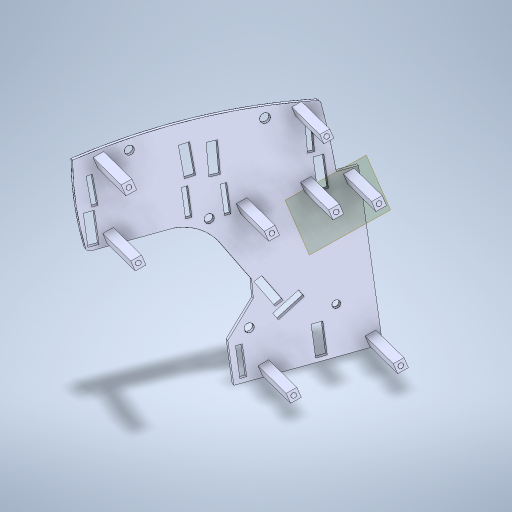
# Autodesk Inventor part: Back Locking Plate - Copy
Saved by Autodesk Inventor 2023 (Build 270158000, 158)
## iProperties
Created: 2022-06-21
Part Number: Back Locking Plate - Copy
Material: Generic
Document SubType Name: Modeling
Designer: Viking Robotics
Density: 1 g/cm^3
Appearance: Default
Sending System: SolidWorks 2019
Last Author: Mahdi
Last Saved: 2022-06-22
Nomenclature: Locking Plate^Bionic Hand
Part Number: Locking Plate^Bionic Hand
Source: NOT_KNOWN
Definition: UNKNOWN
Author: Viking Robotics
Revision Number: ANY
Autodesk Inventor part; units mm, degrees
ref_plane "YZ Plane" through (0, 0, 0) normal (1, 0, 0) x (0, 1, 0)
ref_plane "XZ Plane" through (0, 0, 0) normal (0, 1, 0) x (-1, 0, 0)
ref_plane "XY Plane" through (0, 0, 0) normal (0, 0, 1) x (1, 0, 0)
ref_plane "Work Plane1" through (33.7996, 98.7584, 64.8553) normal (-0.8982078, -0.208723, -0.3868559) x (-0.3186618, -0.2970233, 0.9001288)
sketch "Sketch1" plane through (33.7996, 98.7584, 64.8553) normal (-0.8982078, -0.208723, -0.3868559) x (-0.3186618, -0.2970233, 0.9001288)
  arc A0 (-7.7797, 37.2562) -> (-8.548, 35.9468) centre (-7.048, 35.9468) ccw projected
  arc A1 (73.401, 61.9277) -> (-7.7797, 37.2562) centre (99.9054, -171.1811) ccw
  arc A2 (81.3006, 30.494) -> (73.401, 61.9277) centre (-35.2667, 17.9089) ccw
  arc A3 (-7.7797, 37.2562) -> (-8.548, 35.9468) centre (-7.048, 35.9468) ccw
  arc A4 (-8.548, 35.9468) -> (10.4046, -36.8802) centre (326.4078, 84.2366) ccw
  line L0 (15.9733, -35.39) -> (12.1475, -36.4138) projected
  line L1 (10.4046, -36.8802) -> (15.9733, -35.39)
  line L2 (19.5666, -48.8176) -> (15.9733, -35.39) projected
  line L3 (15.9733, -35.39) -> (19.5666, -48.8176)
  line L4 (55.0191, -39.3303) -> (19.5666, -48.8176) projected
  line L5 (19.5666, -48.8176) -> (55.0191, -39.3303)
  line L6 (37.6609, -14.8207) -> (50.8667, -23.8132) projected
  line L7 (55.0191, -39.3303) -> (50.8667, -23.8132)
  line L8 (50.8667, -23.8132) -> (37.6609, -14.8207)
  line L9 (35.6144, -8.3962) -> (37.6609, -14.8207) projected
  line L10 (37.6609, -14.8207) -> (35.6144, -8.3962)
  line L11 (40.4472, 9.6168) -> (35.6144, -8.3962) projected
  line L12 (35.6144, -8.3962) -> (40.4472, 9.6168)
  arc A5 (52.2969, 22.0311) -> (40.4472, 9.6168) centre (58.9658, 3.8029) ccw
  line L13 (52.2969, 22.0311) -> (79.8228, 29.4185)
  arc A6 (79.8228, 29.4185) -> (81.3006, 31.4948) centre (79.3058, 31.3505) ccw projected
  arc A7 (79.8228, 29.4185) -> (81.3006, 30.494) centre (78.5946, 32.659) ccw
  line L14 (-3.3432, 32.1166) -> (-1.249, 32.7909) projected
  line L15 (-3.3432, 32.1166) -> (-1.249, 32.7909)
  line L16 (-1.249, 32.7909) -> (2.1836, 22.1298)
  line L17 (2.1836, 22.1298) -> (0.0894, 21.4556) projected
  line L18 (2.1836, 22.1298) -> (0.0894, 21.4556)
  line L19 (0.0894, 21.4556) -> (-3.3432, 32.1166)
  line L20 (30.2679, 27.1829) -> (32.3931, 27.7516) projected
  line L21 (30.2679, 27.1829) -> (32.3931, 27.7516)
  line L22 (35.2884, 16.9323) -> (33.1631, 16.3636) projected
  line L23 (32.3931, 27.7516) -> (35.2884, 16.9323)
  line L24 (35.2884, 16.9323) -> (33.1631, 16.3636)
  line L25 (33.1631, 16.3636) -> (30.2679, 27.1829)
  line L26 (42.3754, 33.0619) -> (44.5006, 33.6306) projected
  line L27 (42.3754, 33.0619) -> (44.5006, 33.6306)
  line L28 (44.5006, 33.6306) -> (47.3959, 22.8113)
  line L29 (47.3959, 22.8113) -> (45.2707, 22.2426) projected
  line L30 (47.3959, 22.8113) -> (45.2707, 22.2426)
  line L31 (45.2707, 22.2426) -> (42.3754, 33.0619)
  line L32 (-2.5787, 18.9106) -> (1.0254, 19.8751) projected
  line L33 (-2.5787, 18.9106) -> (1.0254, 19.8751)
  line L34 (1.0254, 19.8751) -> (4.1792, 8.0898) projected
  line L35 (1.0254, 19.8751) -> (4.1792, 8.0898)
  line L36 (4.1792, 8.0898) -> (0.5751, 7.1253) projected
  line L37 (4.1792, 8.0898) -> (0.5751, 7.1253)
  line L38 (0.5751, 7.1253) -> (-2.5787, 18.9106) projected
  line L39 (0.5751, 7.1253) -> (-2.5787, 18.9106)
  line L40 (71.8116, 42.8988) -> (69.3765, 53.8309) projected
  line L41 (69.3765, 53.8309) -> (71.5239, 54.3092) projected
  line L42 (69.3765, 53.8309) -> (71.5239, 54.3092)
  line L43 (71.5239, 54.3092) -> (73.9589, 43.3771) projected
  line L44 (71.5239, 54.3092) -> (73.9589, 43.3771)
  line L45 (73.9589, 43.3771) -> (71.8116, 42.8988) projected
  line L46 (73.9589, 43.3771) -> (71.8116, 42.8988)
  line L47 (71.8116, 42.8988) -> (69.3765, 53.8309)
  line L48 (73.5662, 41.9262) -> (76.1531, 42.6185) projected
  line L49 (76.6566, 30.124) -> (73.5662, 41.9262) projected
  line L50 (73.5662, 41.9262) -> (76.6566, 30.124)
  line L51 (76.6566, 30.124) -> (80.2494, 31.0854)
  line L52 (79.3069, 30.8332) -> (76.6566, 30.124) projected
  line L53 (19.8891, -34.5492) -> (23.7931, -33.5045) projected
  line L54 (19.8891, -34.5492) -> (23.7931, -33.5045)
  line L55 (23.7931, -33.5045) -> (26.9211, -45.1932)
  line L56 (26.9211, -45.1932) -> (23.017, -46.2379) projected
  line L57 (26.9211, -45.1932) -> (23.017, -46.2379)
  line L58 (23.017, -46.2379) -> (19.8891, -34.5492)
  line L59 (46.989, -27.5042) -> (49.2919, -26.8879)
  line L60 (49.1143, -26.9355) -> (52.1388, -38.2378) projected
  line L61 (49.2919, -26.8879) -> (52.3291, -38.2378)
  line L62 (52.3291, -38.2378) -> (50.0136, -38.8065)
  line L63 (52.1388, -38.2378) -> (50.0136, -38.8065) projected
  line L64 (23.0049, -20.2441) -> (33.8224, -23.1464) projected
  line L65 (33.8224, -23.1464) -> (33.0709, -25.9473) projected
  line L66 (23.0049, -20.2441) -> (33.8224, -23.1464)
  line L67 (33.8224, -23.1464) -> (32.9977, -26.22)
  line L68 (32.9977, -26.22) -> (22.1803, -23.3178)
  line L69 (22.2535, -23.045) -> (23.0049, -20.2441) projected
  line L70 (22.1803, -23.3178) -> (23.0049, -20.2441)
  line L71 (32.1159, -9.0624) -> (28.9804, -20.7491)
  line L72 (28.9804, -20.7491) -> (32.1529, -21.2981)
  line L73 (32.1529, -21.2981) -> (35.2884, -9.6114)
  line L74 (35.2884, -9.6114) -> (32.1159, -9.0624)
  line L75 (31.1079, 30.9176) -> (27.3688, 42.5305) projected
  line L76 (33.6535, 31.7372) -> (31.1079, 30.9176) projected
  line L77 (27.3688, 42.5305) -> (31.1079, 30.9176)
  line L78 (31.1079, 30.9176) -> (34.8319, 32.1166)
  line L79 (34.8319, 32.1166) -> (31.0928, 43.7295)
  line L80 (27.3688, 42.5305) -> (29.9144, 43.3501) projected
  line L81 (31.0928, 43.7295) -> (27.3688, 42.5305)
  line L82 (37.1548, 47.166) -> (39.8044, 47.7562) projected
  line L83 (39.8044, 47.7562) -> (42.4321, 35.9592)
  line L84 (42.4321, 35.9592) -> (38.6138, 35.1087)
  line L85 (38.6138, 35.1087) -> (35.9861, 46.9057)
  line L86 (35.9861, 46.9057) -> (39.8044, 47.7562)
  line L87 (50.0136, -38.8065) -> (46.989, -27.5042) projected
  line L88 (50.0136, -38.8065) -> (46.989, -27.5042)
  line L89 (46.989, -27.5042) -> (49.2919, -26.8879)
  line L90 (73.5662, 41.9262) -> (76.6566, 30.124)
  line L91 (80.416, 31.1513) -> (77.2675, 42.9167)
  line L92 (77.2675, 42.9167) -> (73.5662, 41.9262)
  line L93 (-1.249, 32.7909) -> (2.1836, 22.1298)
  line L94 (2.1836, 22.1298) -> (-0.1038, 21.3934)
  line L95 (-0.1038, 21.3934) -> (-3.5364, 32.0544)
  line L96 (-3.5364, 32.0544) -> (-1.249, 32.7909)
  line L97 (73.5662, 41.9262) -> (77.2675, 42.9167)
  line L98 (80.416, 31.1513) -> (76.6566, 30.124)
  circle A8 centre (40.3107, 18.6681) radius 1.7512
  circle A9 centre (42.8297, -23.5628) radius 1.75 projected
  circle A10 centre (42.8297, -23.5628) radius 1.75
  circle A11 centre (13.5965, -31.5233) radius 1.5 projected
  circle A12 centre (13.5965, -31.5233) radius 1.5
  circle A13 centre (10.2348, 41.0072) radius 1.8651
  circle A14 centre (55.1337, 54.975) radius 1.7363
  line L99 (19.5666, -48.8176) -> (4.1792, -52.9353)
  line L100 (4.1792, -52.9353) -> (-16.9374, 17.2047)
  line L101 (-16.9374, 17.2047) -> (-6.3791, 22.7532)
  point P0 (-18.274, -94.7761)
  point P1 (79.8228, 29.4185)
  point P2 (80.6458, 29.8658)
  point P3 (81.2555, 30.9048)
  point P4 (29.9144, 43.3501)
  point P5 (-3.3432, 32.1166)
  point P6 (0.0894, 21.4556)
  point P7 (76.1531, 42.6185)
  point P8 (33.0709, -25.9473)
  constraints: 135 end point, 29 perpendicular, 23 collinear, 14 point on circle, 11 centre point, 2 coincident, 2 parallel, 1 concentric, 1 point on line
extrude "Extrusion1" add sketch "Sketch1" along normal blind 1.5 contours A1 A2 A6 A7 L13 A5 L11 L9 L6 L7 L4 L2 L0 L1 A4 A0
sketch "Sketch2" plane through (42.3456, 47.4595, 72.6908) normal (0.386102, 0.0460551, -0.9213057) x (-0.8982078, -0.208723, -0.3868559)
  line L0 (1.5, 13.9) -> (1.5, 0) projected
  line L1 (0, 13.9) -> (1.5, 13.9)
  line L2 (1.5, 13.9) -> (1.5, 0)
  line L3 (1.5, 0) -> (0, 0)
  line L4 (0, 0) -> (0, 13.9)
  point P0 (76.0619, -34.6143)
  constraints: 8 end point, 2 parallel, 1 horizontal, 1 perpendicular
extrude "Extrusion2" add sketch "Sketch2" along normal blind 15
sketch "Sketch3" plane through (41.6507, 61.3038, 66.8346) normal (-0.2101143, 0.9768898, -0.0392213) x (0.8982078, 0.208723, 0.3868559)
  line L0 (0, -42.4647) -> (0, 9.2353) projected
  line L1 (-1.5, -42.4647) -> (-1.5, 9.2353) projected
  line L2 (0, 9.2353) -> (-1.5, 9.2353)
  line L3 (-1.5, 9.2353) -> (-1.5, -0.6137)
  line L4 (-1.5, -0.6137) -> (0, -0.6137)
  line L5 (0, -0.6137) -> (0, 9.2353)
  point P0 (-76.0619, 42.6703)
  point P1 (-1.5, 9.2353)
  point P2 (0, -0.6137)
  constraints: 8 end point, 2 parallel, 1 horizontal, 1 perpendicular, 1 point on line
extrude "Extrusion3" add sketch "Sketch3" along normal blind 50
sketch "Sketch5" plane through (33.7996, 98.7584, 64.8553) normal (0.8982078, 0.208723, 0.3868559) x (0.3186618, 0.2970233, -0.9001288)
  circle A0 centre (-64.9477, 56.9578) radius 1
  line L0 (-66.9477, 59.1407) -> (-62.9477, 59.1407)
  line L1 (-62.9477, 59.1407) -> (-62.9477, 54.7749)
  line L2 (-62.9477, 54.7749) -> (-66.9477, 54.7749)
  line L3 (-66.9477, 54.7749) -> (-66.9477, 59.1407)
  line L4 (-66.9477, 59.1407) -> (-62.9477, 54.7749) construction
  line L5 (-62.9477, 59.1407) -> (-66.9477, 54.7749) construction
  point P0 (18.274, -94.7761)
  dimension "d24" = 2
  dimension "d25" = 4
  constraints: 12 end point, 2 midpoint, 2 parallel, 1 centre point, 1 horizontal, 1 perpendicular
  measures "d24" diameter of A0
  measures "d25" distance of L1.end L2.end
extrude "Extrusion5" add sketch "Sketch5" along normal blind 25
sketch "Sketch6" plane through (33.7996, 98.7584, 64.8553) normal (0.8982078, 0.208723, 0.3868559) x (0.3186618, 0.2970233, -0.9001288)
  circle A0 centre (-72.1502, 30.9578) radius 1
  circle A1 centre (-64.9477, 56.9578) radius 1 projected
  line L0 (-74.1502, 32.9578) -> (-70.1502, 32.9578)
  line L1 (-70.1502, 32.9578) -> (-70.1502, 28.9578)
  line L2 (-70.1502, 28.9578) -> (-74.1502, 28.9578)
  line L3 (-74.1502, 28.9578) -> (-74.1502, 32.9578)
  line L4 (-74.1502, 32.9578) -> (-70.1502, 28.9578) construction
  line L5 (-70.1502, 32.9578) -> (-74.1502, 28.9578) construction
  point P0 (18.274, -94.7761)
  dimension "d28" = 2
  dimension "d29" = 26
  dimension "d30" = 4
  dimension "d31" = 4
  constraints: 12 end point, 2 midpoint, 2 parallel, 1 centre point, 1 horizontal, 1 perpendicular
  measures "d28" diameter of A0
  measures "d29" vertical distance of A1.centre A0.centre
  measures "d30" distance of L1.end L2.end
  measures "d31" distance of L0.end L1.end
extrude "Extrusion6" add sketch "Sketch6" along normal blind 25 contours L0 L1 L2 L3
sketch "Sketch7" plane through (33.7996, 98.7584, 64.8553) normal (0.8982078, 0.208723, 0.3868559) x (0.3186618, 0.2970233, -0.9001288)
  circle A0 centre (1.0523, 37.9393) radius 1
  circle A1 centre (-64.9477, 56.9578) radius 1 projected
  line L0 (-0.7977, 39.7893) -> (2.9023, 39.7893)
  line L1 (2.9023, 39.7893) -> (2.9023, 36.0893)
  line L2 (2.9023, 36.0893) -> (-0.7977, 36.0893)
  line L3 (-0.7977, 36.0893) -> (-0.7977, 39.7893)
  line L4 (-0.7977, 39.7893) -> (2.9023, 36.0893) construction
  line L5 (2.9023, 39.7893) -> (-0.7977, 36.0893) construction
  point P0 (18.274, -94.7761)
  dimension "d34" = 2
  dimension "d35" = 66
  dimension "d36" = 3.7
  dimension "d37" = 3.7
  constraints: 12 end point, 2 midpoint, 2 parallel, 1 centre point, 1 horizontal, 1 perpendicular
  measures "d34" diameter of A0
  measures "d35" horizontal distance of A1.centre A0.centre
  measures "d36" distance of L1.end L2.end
  measures "d37" distance of L0.end L1.end
extrude "Extrusion7" add sketch "Sketch7" along normal blind 25 contours L0 L1 L2 L3
sketch "Sketch8" plane through (33.7996, 98.7584, 64.8553) normal (0.8982078, 0.208723, 0.3868559) x (0.3186618, 0.2970233, -0.9001288)
  circle A0 centre (-6.1502, 11.9393) radius 1
  circle A1 centre (1.0523, 37.9393) radius 1 projected
  circle A2 centre (-72.1502, 30.9578) radius 1 projected
  line L0 (-8.1502, 13.9393) -> (-4.1502, 13.9393)
  line L1 (-4.1502, 13.9393) -> (-4.1502, 9.9393)
  line L2 (-4.1502, 9.9393) -> (-8.1502, 9.9393)
  line L3 (-8.1502, 9.9393) -> (-8.1502, 13.9393)
  line L4 (-8.1502, 13.9393) -> (-4.1502, 9.9393) construction
  line L5 (-4.1502, 13.9393) -> (-8.1502, 9.9393) construction
  point P0 (18.274, -94.7761)
  dimension "d40" = 2
  dimension "d41" = 26
  dimension "d42" = 66
  dimension "d43" = 4
  dimension "d44" = 4
  constraints: 12 end point, 2 midpoint, 2 parallel, 1 centre point, 1 horizontal, 1 perpendicular
  measures "d40" diameter of A0
  measures "d41" vertical distance of A1.centre A0.centre
  measures "d42" horizontal distance of A2.centre A0.centre
  measures "d43" distance of L1.end L2.end
  measures "d44" distance of L0.end L1.end
extrude "Extrusion8" add sketch "Sketch8" along normal blind 25 contours L0 L1 L2 L3
sketch "Sketch9" plane through (33.7996, 98.7584, 64.8553) normal (0.8982078, 0.208723, 0.3868559) x (0.3186618, 0.2970233, -0.9001288)
  circle A0 centre (-7.199, -49.0216) radius 1
  line L0 (-5.0765, -52.6952) -> (11.4422, 9.0328) projected
  line L1 (-55.0191, -39.3303) -> (-5.0765, -52.6952) projected
  line L2 (-9.199, -47.0216) -> (-5.199, -47.0216)
  line L3 (-5.199, -47.0216) -> (-5.199, -51.0216)
  line L4 (-5.199, -51.0216) -> (-9.199, -51.0216)
  line L5 (-9.199, -51.0216) -> (-9.199, -47.0216)
  line L6 (-9.199, -47.0216) -> (-5.199, -51.0216) construction
  line L7 (-5.199, -47.0216) -> (-9.199, -51.0216) construction
  point P0 (18.274, -94.7761)
  dimension "d47" = 2
  dimension "d48" = 3
  dimension "d49" = 3
  dimension "d50" = 4
  dimension "d51" = 4
  constraints: 12 end point, 2 midpoint, 2 parallel, 1 centre point, 1 horizontal, 1 perpendicular
  measures "d47" diameter of A0
  measures "d48" distance from line of L0 A0.centre
  measures "d49" distance from line of L1 A0.centre
  measures "d50" distance of L3.end L4.end
  measures "d51" distance of L2.end L3.end
extrude "Extrusion9" add sketch "Sketch9" along normal blind 25
sketch "Sketch10" plane through (33.7996, 98.7584, 64.8553) normal (0.8982078, 0.208723, 0.3868559) x (0.3186618, 0.2970233, -0.9001288)
  circle A0 centre (7.7869, 6.9784) radius 1
  line L0 (-5.0765, -52.6952) -> (11.4422, 9.0328) projected
  circle A1 centre (-7.199, -49.0216) radius 1 projected
  line L1 (5.7869, 8.9784) -> (9.7869, 8.9784)
  line L2 (9.7869, 8.9784) -> (9.7869, 4.9784)
  line L3 (9.7869, 4.9784) -> (5.7869, 4.9784)
  line L4 (5.7869, 4.9784) -> (5.7869, 8.9784)
  line L5 (5.7869, 8.9784) -> (9.7869, 4.9784) construction
  line L6 (9.7869, 8.9784) -> (5.7869, 4.9784) construction
  point P0 (18.274, -94.7761)
  dimension "d54" = 2
  dimension "d55" = 3
  dimension "d56" = 56
  dimension "d57" = 4
  dimension "d58" = 4
  constraints: 12 end point, 2 midpoint, 2 parallel, 1 centre point, 1 horizontal, 1 perpendicular
  measures "d54" diameter of A0
  measures "d55" distance from line of L0 A0.centre
  measures "d56" vertical distance of A1.centre A0.centre
  measures "d57" distance of L2.end L3.end
  measures "d58" distance of L1.end L2.end
extrude "Extrusion10" add sketch "Sketch10" along normal blind 25 contours L1 L2 L3 L4
sketch "Sketch11" plane through (33.7996, 98.7584, 64.8553) normal (0.8982078, 0.208723, 0.3868559) x (0.3186618, 0.2970233, -0.9001288)
  circle A0 centre (-43.199, -39.3879) radius 1
  line L0 (-55.0191, -39.3303) -> (-5.0765, -52.6952) projected
  circle A1 centre (-7.199, -49.0216) radius 1 projected
  line L1 (-45.199, -37.3879) -> (-41.199, -37.3879)
  line L2 (-41.199, -37.3879) -> (-41.199, -41.3879)
  line L3 (-41.199, -41.3879) -> (-45.199, -41.3879)
  line L4 (-45.199, -41.3879) -> (-45.199, -37.3879)
  line L5 (-45.199, -37.3879) -> (-41.199, -41.3879) construction
  line L6 (-41.199, -37.3879) -> (-45.199, -41.3879) construction
  point P0 (18.274, -94.7761)
  dimension "d61" = 2
  dimension "d62" = 3
  dimension "d63" = 36
  dimension "d64" = 4
  dimension "d65" = 4
  constraints: 12 end point, 2 midpoint, 2 parallel, 1 centre point, 1 horizontal, 1 perpendicular
  measures "d61" diameter of A0
  measures "d62" distance from line of L0 A0.centre
  measures "d63" horizontal distance of A1.centre A0.centre
  measures "d64" distance of L2.end L3.end
  measures "d65" distance of L1.end L2.end
extrude "Extrusion11" add sketch "Sketch11" along normal blind 25 contours L1 L2 L3 L4
sketch "Sketch12" plane through (33.7996, 98.7584, 64.8553) normal (0.8982078, 0.208723, 0.3868559) x (0.3186618, 0.2970233, -0.9001288)
  circle A0 centre (-28.2131, 16.6121) radius 1
  circle A1 centre (-43.199, -39.3879) radius 1 projected
  circle A2 centre (7.7869, 6.9784) radius 1 projected
  line L0 (-30.2131, 18.6121) -> (-26.2131, 18.6121)
  line L1 (-26.2131, 18.6121) -> (-26.2131, 14.6121)
  line L2 (-26.2131, 14.6121) -> (-30.2131, 14.6121)
  line L3 (-30.2131, 14.6121) -> (-30.2131, 18.6121)
  line L4 (-30.2131, 18.6121) -> (-26.2131, 14.6121) construction
  line L5 (-26.2131, 18.6121) -> (-30.2131, 14.6121) construction
  point P0 (18.274, -94.7761)
  dimension "d68" = 2
  dimension "d69" = 56
  dimension "d70" = 36
  dimension "d71" = 4
  dimension "d72" = 4
  constraints: 12 end point, 2 midpoint, 2 parallel, 1 centre point, 1 horizontal, 1 perpendicular
  measures "d68" diameter of A0
  measures "d69" vertical distance of A1.centre A0.centre
  measures "d70" horizontal distance of A2.centre A0.centre
  measures "d71" distance of L1.end L2.end
  measures "d72" distance of L0.end L1.end
extrude "Extrusion12" add sketch "Sketch12" along normal blind 25 contours L0 L1 L2 L3
body "Solid1"
